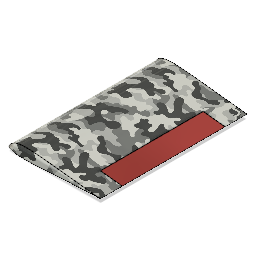
first Wing v1 (Autodesk Fusion 360 design; units mm, degrees)
Autodesk Fusion 360 part; units mm, degrees
sketch "Sketch1" plane through (0, 0, 0) normal (0, 0, 1) x (1, 0, 0)
  line L0 (-55, 0) -> (70, 0)
  spline S0 degree 5 poles (-55, 0) (-54.3189, 1.3622) (-52.723, 3.8251) (-49.6281, 6.7346) (-44.1268, 9.1467) (-35.105, 10.2397) (-24.126, 10.0168) (-11.4291, 8.9792) (2.7201, 7.4687) (18.0816, 5.7136) (34.4618, 3.8474) (48.2736, 2.3192) (58.9972, 1.1633) (66.3058, 0.3885) (70, 0) knots 0 0 0 0 0 0 0.1 0.2 0.3 0.4 0.5 0.6 0.7 0.8 0.9 1 1 1 1 1 1
  line L1 (-60, -10) -> (-50, 10)
  spline S1 degree 5 poles (-55, 0) (-54.8323, -0.6802) (-54.0823, -1.9276) (-51.7151, -3.4602) (-46.0184, -4.8118) (-34.7749, -5.3706) (-19.9417, -4.9258) (-3.5661, -3.9862) (12.9633, -2.9055) (28.8861, -1.8836) (43.8108, -1.0287) (54.8491, -0.5108) (62.619, -0.2186) (67.5767, -0.0659) (70, 0) knots 0 0 0 0 0 0 0.1 0.2 0.3 0.4 0.5 0.6 0.7 0.8 0.9 1 1 1 1 1 1
  line L2 (-39.9719, -5.4464) -> (-10.0281, -4.5536)
  point P0 (-30, 10)
  point P1 (-25, -5)
  dimension "d1" = 125
  dimension "d2" = 5
  constraint horizontal L0
  constraint midpoint L0.start L1
  constraint midpoint P1 L2
  measures "d1" distance of L0.start L0.end
  measures "d2" distance of L0 P1
extrude "Extrude1" add sketch "Sketch1" along normal blind 200 makes body 1
sketch "Sketch2" plane through (0, 0, 0) normal (0, 1, 0) x (1, 0, 0)
  line L0 (70, -170) -> (40, -170)
  line L1 (40, -170) -> (40, -30)
  line L2 (40, -30) -> (70, -30)
  line L3 (70, -30) -> (70, -170)
  line L4 (-55, 0) -> (70, 0)
  line L5 (-55, 0) -> (-55, -200)
  point P0 (70, -200)
  dimension "d6" = 30
  dimension "d7" = 30
  dimension "d8" = 95
  dimension "d9" = 125
  constraint horizontal L0
  constraint perpendicular L0 L1
  constraint perpendicular L1 L2
  constraint perpendicular L0 L3
  measures "d6" distance of L2 L4
  measures "d7" distance of L0 P0
  measures "d8" distance of L0.end L5
  measures "d9" distance of L3 L5
extrude "Extrude2" cut sketch "Sketch2" along normal up to surface end surface at (49.3149, 2.2164, 66.6667) on bodies 1 bodies 1
extrude "Extrude3" cut sketch "Sketch2" along normal up to surface end surface at (-32.8921, -5.1265, 83.3333) on bodies 1 bodies 1
copy_body "CutPasteBodies1" bodies 1 removing the originals makes body 2 in component "Component"
sketch "Sketch1 (2)" plane through (0, 0, 0) normal (0, 0, 1) x (1, 0, 0) in component "Component'"
  line L0 (40, -1.2687, 30) -> (40, 3.2427, 30)
  line L1 (40, 3.2427, 30) -> (70, 0, 30)
  line L2 (70, 0, 30) -> (40, -1.2687, 30)
  point P0 (40, -1.2687)
  point P1 (40, 3.2427)
  point P2 (70, 0)
extrude "Extrude1'" add sketch "Sketch1 (2)" along normal blind 140 separate body contours L0 L1 L2 in plane through (0, 0, 30) normal (0, 0, 1) makes body 3 in component "Component'"
component "Component" placed x (1, 0, 0) y (0, 1, 0) z (0, 0, 1) at (0, 0, 0)
component "Component'" placed x (1, 0, 0) y (0, 1, 0) z (0, 0, 1) at (0, 0, 0)
